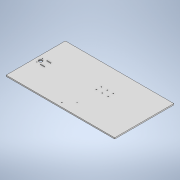
# Autodesk Inventor part: щиток
Saved by Autodesk Inventor 2021.1 (Build 251245010, 245A)
## iProperties
Created: 2023-04-14
Part Number: щиток
Material: Типовые
Document SubType Name: Modeling
Designer: User
Density: 1 g/cm^3
Appearance: По умолчанию
Author: User
Autodesk Inventor part; units mm, degrees
ref_plane "YZ Plane" through (0, 0, 0) normal (1, 0, 0) x (0, 1, 0)
ref_plane "XZ Plane" through (0, 0, 0) normal (0, 1, 0) x (-1, 0, 0)
ref_plane "XY Plane" through (0, 0, 0) normal (0, 0, 1) x (1, 0, 0)
sketch "Эскиз1" plane through (0, 0, 0) normal (0, 1, 0) x (-1, 0, 0)
  ellipse E0 centre (50, 0) end of major axis (50, -150) minor radius 275
  line L0 (50, 150) -> (-225, 150)
  line L1 (-225, 150) -> (-225, -150)
  line L2 (-225, -150) -> (50, -150)
  line L3 (50, -150) -> (50, 150)
  line L4 (50, 150) -> (325, 150)
  line L5 (325, 150) -> (325, -150)
  line L6 (325, -150) -> (50, -150)
  line L7 (50, -150) -> (50, 150)
  point P0 (0, 0)
  point P1 (50, -150)
  point P2 (50, 0)
  dimension "d0" = 275
  dimension "d1" = 150
  dimension "d40" = 325
  constraints: 16 end point, 4 horizontal, 4 parallel, 2 perpendicular, 2 vertical, 1 collinear, 1 horizontal alignment, 1 midpoint, 1 vertical alignment, 2 other
  measures "d40" distance from line of point (0, 0) L5
extrude "Выдавливание1" add sketch "Эскиз1" along normal blind 6
sketch "Эскиз2" plane through (0, 0, 0) normal (0, -1, 0) x (1, 0, 0)
  line L0 (-325, 0) -> (325, 0) construction
  line L1 (225, 150) -> (225, -150) projected
  line L2 (-325, 25) -> (-295, 14.0809)
  line L3 (-295, 14.0809) -> (97.2224, 27.7776)
  line L4 (97.2224, 27.7776) -> (125, 0)
  line L5 (-325, -150) -> (-325, 150) projected
  line L6 (-325, -25) -> (-295, -14.0809)
  line L7 (-295, -14.0809) -> (97.2224, -27.7776)
  line L8 (97.2224, -27.7776) -> (125, 0)
  line L9 (-325, 115) -> (-325, -115)
  line L10 (-260, 60) -> (-190, 60)
  line L11 (-190, 60) -> (-190, 130)
  line L12 (-190, 130) -> (-260, 130)
  line L13 (-260, 130) -> (-260, 60)
  line L14 (-190, 60) -> (-175.5025, 95)
  line L15 (-175.5025, 95) -> (-190, 130)
  line L16 (-218.335, 0) -> (-218.335, 60) construction
  line L17 (-325, 150) -> (225, 150) projected
  line L18 (-325, 150) -> (225, 150) projected
  line L19 (-250, 190) -> (-331.0569, 190) construction
  line L20 (-218.335, 130) -> (-218.335, 190) construction
  line L21 (-175.5025, 51.7755) -> (-260, 130) construction
  line L22 (-260, 60) -> (-175.5025, 138.2245) construction
  circle A0 centre (-222.1933, 95) radius 14.4069 construction
  line L23 (-187.9955, 133) -> (-263, 133)
  line L24 (-263, 133) -> (-263, 57)
  line L25 (-263, 57) -> (-187.9955, 57)
  line L26 (-187.9955, 133) -> (-172.2553, 95)
  line L27 (-172.2553, 95) -> (-187.9955, 57)
  line L28 (-260, 95) -> (-253, 95)
  circle A1 centre (-253, 95) radius 5
  circle A2 centre (-253, 96.75) radius 0.75
  circle A3 centre (-253, 93.25) radius 0.75
  line L29 (-253, 93.25) -> (-253, 96.75)
  point P0 (-331.0569, 190)
  dimension "d5" = 45
  dimension "d8" = 133
  dimension "d9" = 25
  dimension "d10" = 70
  dimension "d12" = 135
  dimension "d13" = 70
  dimension "d16" = 3
  dimension "d17" = 3
  dimension "d20" = 7
  dimension "d21" = 10
  dimension "d27" = 200
  dimension "d35" = 95
  dimension "d36" = 62
  dimension "d37" = 1.75
  dimension "d38" = 1.5
  dimension "d39" = 392.2224
  constraints: 50 end point, 8 point on line, 6 symmetric about line, 4 centre point, 4 equal length, 3 midpoint, 3 parallel, 2 horizontal, 2 perpendicular, 2 vertical, 1 coincident, 1 collinear, 12 other
  measures "d5" angle of L4 L0
  measures "d8" angle of L4 L3
  measures "d9" distance from line of L2.start L0
  measures "d10" angle of L5 L2
  measures "d12" angle of L15 L14
  measures "d13" distance of L11.end L12.end
  measures "d16" distance between parallel lines of L26 L15
  measures "d17" distance between parallel lines of L23 L12
  measures "d20" distance from line of L28.end L13
  measures "d21" diameter of A1
  measures "d36" distance between parallel lines of L5 L24
  measures "d37" distance of A1.centre L29.end
  measures "d38" diameter of A2
  measures "d39" horizontal distance of L3.end L2.end
extrude "Выдавливание2" cut sketch "Эскиз2" against normal blind 0.5
sketch "Эскиз3" plane through (0, 0, 0) normal (0, -1, 0) x (1, 0, 0)
  line L0 (-295, -14.0809) -> (-325, -25) projected
  circle A0 centre (-300.125, 0) radius 8.5
  line L1 (97.2224, -27.7776) -> (-295, -14.0809) projected
  line L2 (-295, -14.0809) -> (-300.125, 0) construction
  circle A1 centre (-305.205, -14.48) radius 1.6
  line L3 (-325, -25) -> (-325, 25) projected
  line L4 (-325, 0) -> (327.0887, 0) construction
  line L5 (-308.505, -17.78) -> (-264.055, -17.78)
  line L6 (-264.055, -17.78) -> (-264.055, 17.78)
  line L7 (-264.055, 17.78) -> (-308.505, 17.78)
  line L8 (-308.505, 17.78) -> (-308.505, -17.78)
  line L9 (-264.055, -17.78) -> (-280.3762, 0) construction
  line L10 (-264.055, 17.78) -> (-280.3762, 0) construction
  line L11 (-264.055, 17.78) -> (-285.037, 17.78)
  line L12 (-285.037, 17.78) -> (-285.037, 14.418)
  line L13 (-285.037, 14.418) -> (-264.055, 14.418)
  line L14 (-264.055, 14.418) -> (-264.055, 17.78)
  line L15 (-285.037, -17.78) -> (-285.037, -14.418)
  line L16 (-285.037, -14.418) -> (-264.055, -14.418)
  circle A2 centre (-305.205, 14.48) radius 1.6
  point P0 (0, 0)
  point P1 (-308.505, 1.4232)
  point P2 (-308.505, -1.4232)
  dimension "d22" = 17
  dimension "d23" = 5.08
  dimension "d25" = 14.48
  dimension "d26" = 3.2
  dimension "d28" = 44.45
  dimension "d29" = 35.56
  dimension "d30" = 8.38
  dimension "d31" = 3.362
  dimension "d32" = 20.982
  constraints: 28 end point, 4 parallel, 4 perpendicular, 4 symmetric about line, 3 centre point, 2 horizontal, 2 point on line, 1 equal length, 1 midpoint, 1 other
  measures "d22" diameter of A0
  measures "d23" horizontal distance of A1.centre L2.end
  measures "d25" vertical distance of A1.centre L2.end
  measures "d26" diameter of A1
  measures "d28" distance of L6.end L7.end
  measures "d29" distance of L7.end L5.start
  measures "d30" distance from line of L8 L2.end
  measures "d31" distance between parallel lines of L11 L13
  measures "d32" distance between parallel lines of L6 L12
extrude "Выдавливание3" cut sketch "Эскиз3" against normal blind 14.48 contours L15 L16 L6 L1 | L1 L6 L5 L15 | L8 A0 | L13 L12 L7 L6 | A1 | A2 picked at (-298.3314, -3.5155)
sketch "Эскиз4" plane through (0, 0, 0) normal (0, -1, 0) x (1, 0, 0)
  line L0 (0, 0) -> (-4.3, 0) construction
  line L1 (-4.3, 0) -> (-4.3, -50) construction
  line L2 (-4.3, -50) -> (0, -50) construction
  line L3 (0, -50) -> (0, 0) construction
  circle A0 centre (-2.15, -15) radius 2.15
  circle A1 centre (-2.15, -40) radius 2.15
  line L4 (-30, 0) -> (-34.3, 0) construction
  line L5 (-34.3, 0) -> (-34.3, -50) construction
  line L6 (-34.3, -50) -> (-30, -50) construction
  line L7 (-30, -50) -> (-30, 0) construction
  circle A2 centre (-32.15, -15) radius 2.15
  circle A3 centre (-32.15, -40) radius 2.15
  line L8 (30, 0) -> (25.7, 0) construction
  line L9 (25.7, 0) -> (25.7, -50) construction
  line L10 (25.7, -50) -> (30, -50) construction
  line L11 (30, -50) -> (30, 0) construction
  circle A4 centre (27.85, -15) radius 2.15
  circle A5 centre (27.85, -40) radius 2.15
  line L12 (0, 0) -> (-4.3, 0) construction
  line L13 (-4.3, 0) -> (-4.3, -50) construction
  line L14 (-4.3, -50) -> (0, -50) construction
  line L15 (0, -50) -> (0, 0) construction
  circle A6 centre (-2.15, -15) radius 2.15
  circle A7 centre (-2.15, -40) radius 2.15
  circle A8 centre (-63.7357, 129.0861) radius 2.1
  circle A9 centre (-24.6255, 90.6066) radius 1.6
  dimension "d41" = 4.3
  dimension "d42" = 50
  dimension "d43" = 10
  dimension "d44" = 15
  dimension "d47" = 30
  dimension "d50" = 30
  dimension "d53" = 4.2
  dimension "d54" = 3.2
  constraints: 32 end point, 10 centre point, 4 tangent, 3 horizontal, 2 collinear, 2 parallel, 1 perpendicular, 34 other
  measures "d41" distance between parallel lines of L3 L1
  measures "d42" distance between parallel lines of L0 L2
  measures "d43" distance from line of L2 A1.centre
  measures "d44" distance from line of A0.centre L0
  measures "d47" distance of L1.end L5.end
  measures "d50" distance of L1.end L9.end
  measures "d53" diameter of A8
  measures "d54" diameter of A9
extrude "Выдавливание4" cut sketch "Эскиз4" against normal blind 10
equation "\"d33\" = d25"
